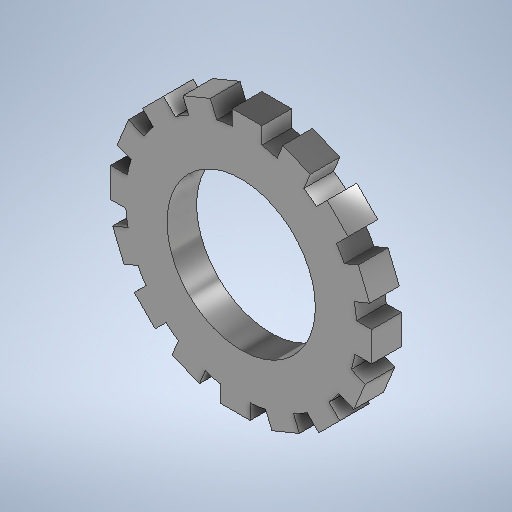
# Autodesk Inventor part: cad@36
Saved by Autodesk Inventor 2025.2 (Build 292293000, 293)
## iProperties
Created: 2025-03-24
Part Number: cad@36
Material: Generic
Document SubType Name: Modeling
Designer: spars
Density: 1 g/cm^3
Appearance: Chrome - Polished Black
Author: spars
Autodesk Inventor part; units mm, degrees
ref_plane "XZ Plane" through (0, 0, 0) normal (0, 1, 0) x (-1, 0, 0)
ref_plane "XY Plane" through (0, 0, 0) normal (0, 0, 1) x (1, 0, 0)
sketch "Sketch1" plane through (0, 0, 0) normal (0, 0, 1) x (1, 0, 0)
  line L0 (-522.2408, 82.6105) -> (-274.5908, 82.6105) construction
  line L1 (-274.5908, 82.6105) -> (-274.5908, -141.3329) construction
  line L2 (-274.5908, -141.3329) -> (-522.2408, -141.3329) construction
  line L3 (-522.2408, -141.3329) -> (-522.2408, 82.6105) construction
  circle A0 centre (0, 0) radius 25
  circle A1 centre (0, 0) radius 39
  dimension "d7" = 50
  dimension "d8" = 78
  constraints: 2 centre point, 2 coincident, 2 other
  measures "d7" diameter of A0
  measures "d8" diameter of A1
extrude "Extrusion1" add sketch "Sketch1" along normal blind 10
ref_plane "Work Plane1" through (39, 0, 0) normal (1, 0, 0) x (0, 1, 0)
sketch "Sketch2" plane through (39, 0, 0) normal (1, 0, 0) x (0, 1, 0)
  line L0 (39, 10) -> (-39, 10) projected
  line L1 (3.0144, 10) -> (-6.9856, 10)
  line L2 (-6.9856, 10) -> (-6.9856, 0)
  line L3 (-6.9856, 0) -> (3.0144, 0)
  line L4 (3.0144, 0) -> (3.0144, 10)
  point P0 (0, 0)
  dimension "d13" = 10
  dimension "d14" = 10
  constraints: 8 end point, 2 parallel, 1 horizontal, 1 perpendicular, 1 point on line
  measures "d13" distance of L3.end L2.end
  measures "d14" distance of L2.end L1.end
extrude "Extrusion2" add sketch "Sketch2" along normal blind 5 and the other way blind 5
pattern_circular "Circular Pattern1" count 16 over 360 about axis through (0, 0, 0) along (0, 0, 1) of "Extrusion2"
body "Solid1"
